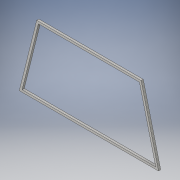
# Autodesk Inventor part: Truss Template
Saved by Autodesk Inventor 2016 (Build 200138000, 138)
## iProperties
Created: 2016-01-30
Part Number: Truss Template
Material: Generic
Document SubType Name: Modeling
Designer: Kurtis
Density: 1 g/cm^3
Appearance: Default
Author: Kurtis
Autodesk Inventor part; units mm, degrees
ref_plane "YZ Plane" through (0, 0, 0) normal (1, 0, 0) x (0, 1, 0)
ref_plane "XZ Plane" through (0, 0, 0) normal (0, 1, 0) x (-1, 0, 0)
ref_plane "XY Plane" through (0, 0, 0) normal (0, 0, 1) x (1, 0, 0)
sketch "Sketch1" plane through (0, 0, 0) normal (0, 0, 1) x (1, 0, 0)
  line L0 (0, 0) -> (203.2, 0)
  line L1 (25.4, 101.6) -> (0, 0)
  line L2 (177.8, 101.6) -> (203.2, 0)
  line L3 (177.8, 101.6) -> (25.4, 101.6)
  line L4 (101.6, 0) -> (76.2, 0) construction
  line L5 (76.2, 0) -> (127, 0) construction
  line L6 (127, 101.6) -> (152.4, 101.6)
  line L7 (25.4, 101.6) -> (50.8, 101.6)
  line L8 (27.879, 98.425) -> (175.321, 98.425)
  line L9 (175.321, 98.425) -> (199.1335, 3.175)
  line L10 (199.1335, 3.175) -> (4.0665, 3.175)
  line L11 (25.4, 101.6) -> (28.575, 101.6) construction
  line L12 (0, 0) -> (3.175, 0) construction
  line L13 (4.0665, 3.175) -> (27.879, 98.425)
  dimension "d0" = 203.2
  dimension "d9" = 152.4
  dimension "d20" = 3.175
  dimension "d21" = 3.175
  dimension "d24" = 3.175
  dimension "d25" = 3.175
  dimension "d35" = 101.6
  constraints: 28 end point, 7 point on line, 3 parallel, 1 equal length, 1 horizontal, 1 midpoint
  measures "d0" distance of L0.start L0.end
  measures "d9" distance of L2.start L1.start
  measures "d20" distance between parallel lines of L13 L1
  measures "d21" distance between parallel lines of L9 L2
  measures "d24" distance between parallel lines of L10 L0
  measures "d25" distance between parallel lines of L3 L8
  measures "d35" vertical distance of L1.start L0.start
extrude "Extrusion1" add sketch "Sketch1" along normal blind 3.175
body "Solid1"
